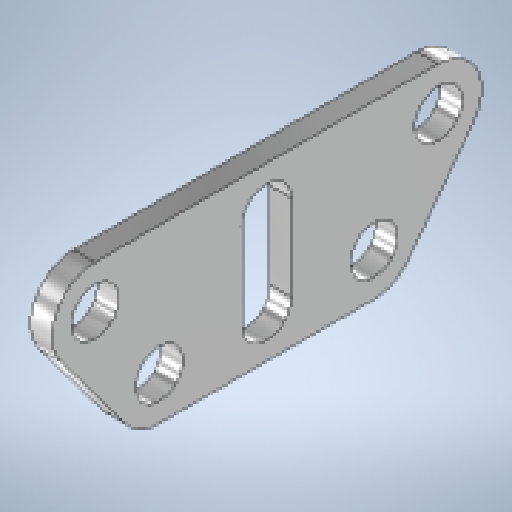
# Autodesk Inventor part: Pin Cap - Slot
Saved by Autodesk Inventor 2023.4 (Build 274418000, 418)
## iProperties
Created: 2024-04-23
Part Number: Pin Cap - Slot
Material: Aluminum 6061
Document SubType Name: Modeling
Designer: Nathan Cai
Density: 2.7 g/cm^3
Appearance: Aluminum - Flat
Author: Nathan Cai
Autodesk Inventor part; units mm, degrees
ref_plane "YZ Plane" through (0, 0, 0) normal (1, 0, 0) x (0, 1, 0)
ref_plane "XZ Plane" through (0, 0, 0) normal (0, 1, 0) x (-1, 0, 0)
ref_plane "XY Plane" through (0, 0, 0) normal (0, 0, 1) x (1, 0, 0)
sketch "Sketch1" plane through (0, 0, 0) normal (1, 0, 0) x (0, 1, 0)
  line L0 (3.175, 0) -> (-3.175, 0) construction
  line L1 (3.175, 1.5875) -> (-3.175, 1.5875) construction
  line L2 (-3.175, -1.5875) -> (3.175, -1.5875) construction
  arc A0 (3.175, -1.5875) -> (3.175, 1.5875) centre (3.175, 0) ccw construction
  arc A1 (-3.175, 1.5875) -> (-3.175, -1.5875) centre (-3.175, 0) ccw construction
  circle A2 centre (3.175, -12.7) radius 1.7526
  circle A3 centre (-3.175, -7.9375) radius 1.7526
  line L3 (3.175, -1.8415) -> (-3.175, -1.8415)
  arc A4 (-3.175, 1.8415) -> (-3.175, -1.8415) centre (-3.175, 0) ccw
  line L4 (-3.175, 1.8415) -> (3.175, 1.8415)
  arc A5 (3.175, -1.8415) -> (3.175, 1.8415) centre (3.175, 0) ccw
  arc A6 (1.27, -15.24) -> (6.35, -12.7) centre (3.175, -12.7) ccw
  arc A7 (-6.35, -7.9375) -> (-5.08, -10.4775) centre (-3.175, -7.9375) ccw
  line L5 (-5.08, -10.4775) -> (1.27, -15.24)
  line L6 (6.35, -12.7) -> (6.35, 0)
  line L7 (-6.35, -7.9375) -> (-6.35, 0)
  circle A8 centre (3.175, 12.7) radius 1.7526
  circle A9 centre (-3.175, 7.9375) radius 1.7526
  arc A10 (6.35, 12.7) -> (1.27, 15.24) centre (3.175, 12.7) ccw
  arc A11 (-5.08, 10.4775) -> (-6.35, 7.9375) centre (-3.175, 7.9375) ccw
  line L8 (-5.08, 10.4775) -> (1.27, 15.24)
  line L9 (6.35, 12.7) -> (6.35, 0)
  line L10 (-6.35, 7.9375) -> (-6.35, 0)
  point P0 (0, 0)
  dimension "d0" = 3.175
  dimension "d1" = 3.175
  dimension "d4" = 3.5052
  dimension "d5" = 12.7
  dimension "d6" = 3.175
  dimension "d7" = 3.5052
  dimension "d8" = 3.175
  dimension "d9" = 4.7625
  dimension "d10" = 0.254
  dimension "d11" = 6.35
  dimension "d12" = 6.35
  constraints: 24 end point, 16 point on circle, 12 centre point, 8 symmetric about line, 8 tangent, 4 coincident, 2 parallel, 2 point on line, 2 vertical, 1 horizontal, 1 midpoint, 7 other
  measures "d0" distance of point (0, 0) L0.end
  measures "d1" diameter of A1
  measures "d4" diameter of A2
  measures "d5" distance from line of L0 A2.centre
  measures "d6" horizontal distance of A2.centre point (0, 0)
  measures "d7" diameter of A3
  measures "d8" horizontal distance of point (0, 0) A3.centre
  measures "d9" vertical distance of A2.centre A3.centre
  measures "d10" distance between parallel lines of L2 L3
  measures "d11" diameter of A6
  measures "d12" diameter of A7
extrude "Extrusion1" add sketch "Sketch1" along normal blind 1.5875
equation "\"d8\" = d6"
body "Solid1"
